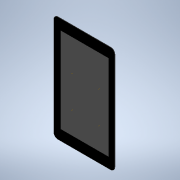
# Autodesk Inventor part: display
Saved by Autodesk Inventor 2021 (Build 250183000, 183)
## iProperties
Created: 2021-07-13
Part Number: display
Material: Generisch
Document SubType Name: Modeling
Designer: Simon
Density: 1 g/cm^3
Appearance: Vorgabe
Author: Simon
Autodesk Inventor part; units mm, degrees
ref_plane "YZ Plane" through (0, 0, 0) normal (1, 0, 0) x (0, 1, 0)
ref_plane "XZ Plane" through (0, 0, 0) normal (0, 1, 0) x (-1, 0, 0)
ref_plane "XY Plane" through (0, 0, 0) normal (0, 0, 1) x (1, 0, 0)
sketch "Skizze1" plane through (0, 0, 0) normal (0, 0, 1) x (1, 0, 0)
  line L0 (-55.5, 96.5) -> (55.5, 96.5)
  line L1 (55.5, 96.5) -> (55.5, -96.5)
  line L2 (55.5, -96.5) -> (-55.5, -96.5)
  line L3 (-55.5, -96.5) -> (-55.5, 96.5)
  point P0 (0, 0)
  point P1 (0, 96.5)
  point P2 (-55.5, 0)
  dimension "d0" = 111
  dimension "d1" = 193
  constraints: 8 end point, 2 midpoint, 2 parallel, 1 horizontal, 1 horizontal alignment, 1 perpendicular, 1 vertical alignment
  measures "d0" distance between parallel lines of L1 L3
  measures "d1" distance between parallel lines of L2 L0
extrude "Extrusion1" add sketch "Skizze1" against normal blind 0.65
sketch "Skizze3" plane through (0, 0, 0) normal (0, 0, 1) x (1, 0, 0)
  line L0 (-42.5, 77.5) -> (44.5, 77.5)
  line L1 (44.5, 77.5) -> (44.5, -77.5)
  line L2 (44.5, -77.5) -> (-42.5, -77.5)
  line L3 (-42.5, -77.5) -> (-42.5, 77.5)
  line L4 (55.5, 96.5) -> (-55.5, 96.5) projected
  line L5 (-55.5, -96.5) -> (55.5, -96.5) projected
  line L6 (-55.5, 96.5) -> (-55.5, -96.5) projected
  point P0 (0, 0)
  dimension "d11" = 155
  dimension "d12" = 19
  dimension "d13" = 19
  dimension "d14" = 87
  dimension "d15" = 13
  constraints: 8 end point, 2 parallel, 1 horizontal, 1 perpendicular
  measures "d11" distance between parallel lines of L2 L0
  measures "d12" distance between parallel lines of L4 L0
  measures "d13" distance between parallel lines of L5 L2
  measures "d14" distance between parallel lines of L3 L1
  measures "d15" distance between parallel lines of L6 L3
split_face "Trennen1"
fillet "Rundung1" radius 7.5 4 edges at (-55.5, -96.5, -0.325) (55.5, -96.5, -0.325) (55.5, 96.5, -0.325) (-55.5, 96.5, -0.325)
sketch "Skizze2" plane through (0, 0, -0.65) normal (0, 0, -1) x (-1, 0, 0)
  line L0 (-49, 81.5) -> (52, 81.5)
  line L1 (52, 81.5) -> (52, -85.5)
  line L2 (52, -85.5) -> (-49, -85.5)
  line L3 (-49, -85.5) -> (-49, 81.5)
  line L4 (55.5, -96.5) -> (55.5, 96.5) projected
  line L5 (55.5, 96.5) -> (-55.5, 96.5) projected
  point P0 (0, 0)
  dimension "d5" = 101
  dimension "d6" = 167
  dimension "d7" = 3.5
  dimension "d8" = 15
  constraints: 8 end point, 2 parallel, 1 horizontal, 1 perpendicular
  measures "d5" distance between parallel lines of L1 L3
  measures "d6" distance between parallel lines of L2 L0
  measures "d7" distance between parallel lines of L1 L4
  measures "d8" distance between parallel lines of L5 L0
extrude "Extrusion2" add sketch "Skizze2" along normal blind 5.1
sketch "Skizze6" plane through (0, 0, -5.75) normal (0, 0, -1) x (-1, 0, 0)
  line L0 (-38, 68.5) -> (-30, 68.5)
  line L1 (-30, 68.5) -> (-30, 53.5)
  line L2 (-30, 53.5) -> (-38, 53.5)
  line L3 (-38, 53.5) -> (-38, 68.5)
  line L4 (28, 68.5) -> (36, 68.5)
  line L5 (36, 68.5) -> (36, 53.5)
  line L6 (36, 53.5) -> (28, 53.5)
  line L7 (28, 53.5) -> (28, 68.5)
  line L8 (-38, -57.5) -> (-30, -57.5)
  line L9 (-30, -57.5) -> (-30, -72.5)
  line L10 (-30, -72.5) -> (-38, -72.5)
  line L11 (-38, -72.5) -> (-38, -57.5)
  line L12 (28, -57.5) -> (36, -57.5)
  line L13 (36, -57.5) -> (36, -72.5)
  line L14 (36, -72.5) -> (28, -72.5)
  line L15 (28, -72.5) -> (28, -57.5)
  line L16 (-49, 81.5) -> (-49, -85.5) projected
  line L17 (52, 81.5) -> (-49, 81.5) projected
  line L18 (52, -85.5) -> (52, 81.5) projected
  line L19 (-49, -85.5) -> (52, -85.5) projected
  point P0 (0, 0)
  dimension "d35" = 8
  dimension "d36" = 15
  dimension "d37" = 11
  dimension "d38" = 13
  dimension "d39" = 16
  dimension "d40" = 13
  constraints: 32 end point, 8 parallel, 5 equal length, 4 horizontal, 4 perpendicular, 2 horizontal alignment, 2 point on line, 2 vertical alignment
  measures "d35" distance between parallel lines of L3 L1
  measures "d36" distance between parallel lines of L0 L2
  measures "d37" distance between parallel lines of L16 L3
  measures "d38" distance between parallel lines of L17 L0
  measures "d39" distance between parallel lines of L18 L5
  measures "d40" distance between parallel lines of L19 L10
extrude "Extrusion5" add sketch "Skizze6" along normal blind 2.5 contours L0 L1 L2 L3 | L4 L5 L6 L7 | L8 L9 L10 L11 | L12 L13 L14 L15
sketch "Skizze7" plane through (0, 0, -8.25) normal (0, 0, -1) x (-1, 0, 0)
  line L0 (-30, 68.5) -> (-38, 68.5) projected
  line L1 (-38, 68.5) -> (-38, 53.5) projected
  point P0 (0, 0)
  point P1 (-34, 61)
  point P2 (32, 61)
  point P3 (32, -65.5)
  point P4 (-34, -65.5)
  point P5 (-34, 68.5)
  point P6 (-38, 61)
  dimension "d43" = 126.5
  dimension "d44" = 66
  constraints: 3 horizontal alignment, 3 vertical alignment, 2 midpoint
  measures "d43" distance of point (-34, -65.5) point (-34, 61)
  measures "d44" distance of point (32, -65.5) point (-34, -65.5)
sketch "Skizze8" plane through (38, 53.5, -5.75) normal (1, 0, 0) x (0, 0, -1)
  line L0 (0, 15) -> (2.5, 15) projected
  line L1 (0, 0) -> (2.5, 0) projected
  line L2 (0, -111) -> (2.5, -111) projected
  line L3 (0, -126) -> (2.5, -126) projected
  line L4 (2.5, -111) -> (2.5, -126) projected
  line L5 (0, -111) -> (2.5, -115)
  line L6 (2.5, -111) -> (2.5, -126) projected
  line L7 (0, -126) -> (2.5, -126) projected
  line L8 (0, -126) -> (2.5, -122)
  line L9 (0, 15) -> (0, 0) projected
  line L10 (0, 0) -> (2.5, 4)
  line L11 (2.5, 0) -> (2.5, 15) projected
  line L12 (0, 15) -> (2.5, 15) projected
  line L13 (0, 15) -> (2.5, 11)
  line L14 (0, 28) -> (0, -139) projected
  line L15 (0, 14.0566) -> (2, 10.8566)
  line L16 (2, 10.8566) -> (2, 4.1434)
  line L17 (2, 4.1434) -> (0, 0.9434)
  line L18 (0, -126) -> (0, -111) projected
  line L19 (0, -111.9434) -> (2, -115.1434)
  line L20 (2, -115.1434) -> (2, -121.8566)
  line L21 (2, -121.8566) -> (0, -125.0566)
  point P0 (-5.75, -53.5)
  point P1 (0, -111.9434)
  point P2 (0, 14.0566)
  point P3 (0, 0.9434)
  dimension "d45" = 7
  dimension "d46" = 0.5
  dimension "d47" = 0.5
  dimension "d48" = 0.5
  dimension "d49" = 0.5
  constraints: 20 end point, 7 point on line, 4 equal length, 4 parallel, 1 vertical, 4 other
  measures "d45" distance of L13.end L10.end
  measures "d46" distance between parallel lines of L11 L16
  measures "d47" distance between parallel lines of L13 L15
  measures "d48" distance between parallel lines of L10 L17
  measures "d49" distance between parallel lines of L5 L19
extrude "Extrusion6" cut sketch "Skizze8" along normal through all both and the other way through all contours L2 L4 L5 | L0 L11 L13 | L15 L16 L17 L9 | L11 L1 L10 | L19 L20 L21 L14 | L4 L3 L8
hole "Bohrung1" at (34, 61, -8.25) at (-32, 61, -8.25) at (-32, -65.5, -8.25) at (34, -65.5, -8.25) direction (0, 0, 1) diameter 2.459 depth 0.5 thread size "M3x0.5" class "6H" standard "ISO Metric profile"
sketch "Skizze4" plane through (0, 0, -5.75) normal (0, 0, -1) x (-1, 0, 0)
  line L0 (-31.5, 25) -> (24.5, 25)
  line L1 (24.5, 25) -> (24.5, -40)
  line L2 (24.5, -40) -> (-31.5, -40)
  line L3 (-31.5, -40) -> (-31.5, 25)
  line L4 (-49, -85.5) -> (52, -85.5) projected
  line L5 (-49, 81.5) -> (-49, -85.5) projected
  point P0 (0, 0)
  dimension "d17" = 45.5
  dimension "d18" = 65
  dimension "d19" = 56
  dimension "d20" = 17.5
  constraints: 8 end point, 2 parallel, 1 horizontal, 1 perpendicular
  measures "d17" distance between parallel lines of L4 L2
  measures "d18" distance between parallel lines of L2 L0
  measures "d19" distance between parallel lines of L1 L3
  measures "d20" distance between parallel lines of L5 L3
extrude "Extrusion3" add sketch "Skizze4" along normal blind 3.45
sketch "Skizze5" plane through (0, 0, -9.2) normal (0, 0, -1) x (-1, 0, 0)
  line L0 (-26.8453, -34.5) -> (-25.6906, -36.5)
  line L1 (-25.6906, -36.5) -> (-26.8453, -38.5)
  line L2 (-26.8453, -38.5) -> (-29.1547, -38.5)
  line L3 (-29.1547, -38.5) -> (-30.3094, -36.5)
  line L4 (-30.3094, -36.5) -> (-29.1547, -34.5)
  line L5 (-29.1547, -34.5) -> (-26.8453, -34.5)
  line L6 (-26.8453, 23.5) -> (-25.6906, 21.5)
  line L7 (-25.6906, 21.5) -> (-26.8453, 19.5)
  line L8 (-26.8453, 19.5) -> (-29.1547, 19.5)
  line L9 (-29.1547, 19.5) -> (-30.3094, 21.5)
  line L10 (-30.3094, 21.5) -> (-29.1547, 23.5)
  line L11 (-29.1547, 23.5) -> (-26.8453, 23.5)
  line L12 (22.1547, 23.5) -> (23.3094, 21.5)
  line L13 (23.3094, 21.5) -> (22.1547, 19.5)
  line L14 (22.1547, 19.5) -> (19.8453, 19.5)
  line L15 (19.8453, 19.5) -> (18.6906, 21.5)
  line L16 (18.6906, 21.5) -> (19.8453, 23.5)
  line L17 (19.8453, 23.5) -> (22.1547, 23.5)
  line L18 (22.1547, -34.5) -> (23.3094, -36.5)
  line L19 (23.3094, -36.5) -> (22.1547, -38.5)
  line L20 (22.1547, -38.5) -> (19.8453, -38.5)
  line L21 (19.8453, -38.5) -> (18.6906, -36.5)
  line L22 (18.6906, -36.5) -> (19.8453, -34.5)
  line L23 (19.8453, -34.5) -> (22.1547, -34.5)
  line L24 (24.5, 25) -> (-31.5, 25) projected
  line L25 (-31.5, -40) -> (24.5, -40) projected
  line L26 (24.5, -40) -> (24.5, 25) projected
  line L27 (-31.5, 25) -> (-31.5, -40) projected
  point P0 (0, 0)
  point P1 (-28, -36.5)
  point P2 (-28, 21.5)
  point P3 (21, 21.5)
  point P4 (21, -36.5)
  point P5 (-28, 21.5)
  point P6 (21, 21.5)
  point P7 (21, -36.5)
  point P8 (-28, -36.5)
  dimension "d23" = 4
  dimension "d24" = 4
  dimension "d25" = 4
  dimension "d26" = 4
  dimension "d27" = 49
  dimension "d28" = 58
  dimension "d29" = 65
  dimension "d30" = 3.5
  dimension "d31" = 56
  dimension "d32" = 3.5
  constraints: 48 end point, 4 coincident, 4 horizontal, 2 horizontal alignment, 2 vertical alignment, 52 other
  measures "d23" distance between parallel lines of L0 L3
  measures "d24" distance between parallel lines of L6 L9
  measures "d25" distance between parallel lines of L12 L15
  measures "d26" distance between parallel lines of L18 L21
  measures "d27" distance of point (21, -36.5) point (-28, -36.5)
  measures "d28" distance of point (-28, 21.5) point (-28, -36.5)
  measures "d29" distance between parallel lines of L24 L25
  measures "d30" distance from line of L25 point (-28, -36.5)
  measures "d31" distance between parallel lines of L26 L27
  measures "d32" distance from line of point (21, -36.5) L26
extrude "Extrusion4" add sketch "Skizze5" along normal blind 12 contours L0 L1 L2 L3 L4 L5 | L6 L7 L8 L9 L10 L11 | L12 L13 L14 L15 L16 L17 | L18 L19 L20 L21 L22 L23
equation "\"d47\" = d46"
equation "\"d48\" = d47"
equation "\"d49\" = d48"
equation "\"d30\" = -0.5 * d28 + 0.5 * d29"
equation "\"d32\" = -0.5 * d27 + 0.5 * d31"
